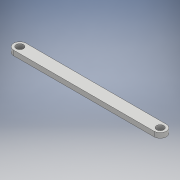
# Autodesk Inventor part: portabateria 2.0
Saved by Autodesk Inventor 2018 (Build 220112000, 112)
## iProperties
Created: 2017-05-13
Part Number: portabateria 2.0
Material: Generic
Document SubType Name: Modeling
Designer: Vidal Villegas
Density: 1 g/cm^3
Appearance: Default
Author: Vidal Villegas
Autodesk Inventor part; units mm, degrees
ref_plane "YZ Plane" through (0, 0, 0) normal (1, 0, 0) x (0, 1, 0)
ref_plane "XZ Plane" through (0, 0, 0) normal (0, 1, 0) x (-1, 0, 0)
ref_plane "XY Plane" through (0, 0, 0) normal (0, 0, 1) x (1, 0, 0)
sketch "Sketch1" plane through (0, 0, 0) normal (0, 0, 1) x (1, 0, 0)
  circle A0 centre (0, 0) radius 1.5
  circle A1 centre (57.756, 0) radius 1.5
  line L0 (0, 2.5) -> (57.756, 2.5)
  line L1 (0, -2.5) -> (57.756, -2.5)
  line L2 (0, 0) -> (0.5, 0) construction
  arc A2 (0, 2.5) -> (0, -2.5) centre (0, 0) ccw
  arc A3 (57.756, -2.5) -> (57.756, 2.5) centre (57.756, 0) ccw
  dimension "d0" = 57.756
  dimension "d1" = 5
  dimension "d2" = 3
  dimension "d3" = 0.5
  constraints: 6 end point, 4 centre point, 4 point on circle, 4 vertical alignment, 3 coincident, 3 horizontal, 1 equal radius, 1 horizontal alignment, 1 other
  measures "d0" distance of A1.centre point (0, 0)
  measures "d1" distance between parallel lines of L1 L0
  measures "d2" diameter of A0
  measures "d3" distance of L2.start L2.end
extrude "Extrusion1" add sketch "Sketch1" along normal blind 2
body "Solid1"
